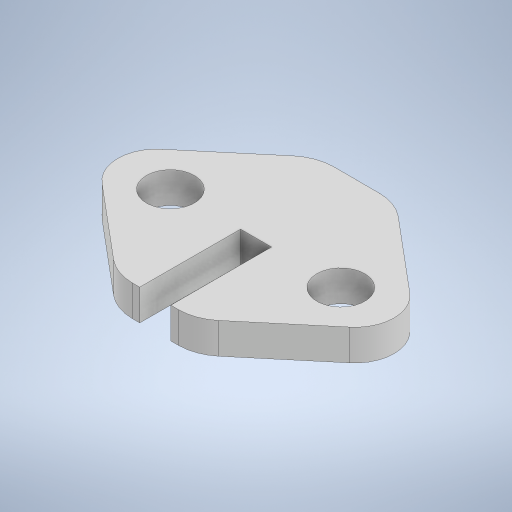
# Autodesk Inventor part: back_lock
Saved by Autodesk Inventor 2024 (Build 280153000, 153)
## iProperties
Created: 2024-04-22
Part Number: back_lock
Material: Generic
Document SubType Name: Modeling
Designer: nikop
Density: 1 g/cm^3
Appearance: Default
Author: nikop
Autodesk Inventor part; units mm, degrees
ref_plane "YZ Plane" through (0, 0, 0) normal (1, 0, 0) x (0, 1, 0)
ref_plane "XZ Plane" through (0, 0, 0) normal (0, 1, 0) x (-1, 0, 0)
ref_plane "XY Plane" through (0, 0, 0) normal (0, 0, 1) x (1, 0, 0)
sketch "Sketch1" plane through (0, 0, 0) normal (0, 1, 0) x (-1, 0, 0)
  line L0 (4.2489, -4.8935) -> (8.8452, -1.0368)
  line L1 (-0.6227, -5.5713) -> (0.8666, -5.5713)
  arc A0 (2.3695, -5.5775) -> (4.2489, -4.8935) centre (2.3418, -2.5777) ccw
  line L2 (0.8803, -5.5773) -> (2.3695, -5.5775)
  arc A1 (-2.502, -4.8873) -> (-0.6227, -5.5713) centre (-0.595, -2.5715) ccw
  circle A2 centre (6.3667, 0.9564) radius 1.55
  arc A3 (8.8452, -1.0368) -> (8.8476, 2.8817) centre (7.2935, 0.9234) ccw
  line L3 (-0.1334, 0.9212) -> (1.8666, 0.9212)
  arc A4 (-0.6442, 7.4287) -> (-2.5236, 6.7446) centre (-0.6165, 4.4288) ccw
  line L4 (-0.6442, 7.4287) -> (-0.1334, 7.4287)
  line L5 (-0.1334, 0.9212) -> (-0.1334, 7.4287)
  line L6 (1.8666, 0.9212) -> (1.8827, 7.4237)
  line L7 (1.8827, 7.4237) -> (2.372, 7.4225)
  arc A5 (4.2514, 6.7384) -> (2.372, 7.4225) centre (2.3443, 4.4226) ccw
  line L8 (4.2514, 6.7384) -> (8.8476, 2.8817)
  line L9 (-2.502, -4.8873) -> (-7.0983, -1.0306)
  line L10 (-2.5236, 6.7446) -> (-7.1199, 2.8879)
  circle A6 centre (-4.6336, 0.9477) radius 1.55
  arc A7 (-7.1199, 2.8879) -> (-7.0983, -1.0306) centre (-5.5563, 0.9372) ccw
  line L11 (0.8803, -5.5773) -> (0.8666, -5.5713)
  point P0 (0, 0)
  dimension "d0" = 2
  dimension "d1" = 3
  dimension "d2" = 2
  dimension "d3" = 3
  dimension "d4" = 2
  dimension "d5" = 3
  dimension "d6" = 2
  dimension "d7" = 3
  dimension "d8" = 3.1
  dimension "d9" = 3.1
  dimension "d10" = 6
  dimension "d11" = 6
  dimension "d12" = 2.5
  dimension "d13" = 6
  dimension "d14" = 6
  dimension "d15" = 2.5
  constraints: 24 end point, 12 point on circle, 8 centre point, 1 horizontal, 1 perpendicular
  measures "d0" distance of L7.end L8.start
  measures "d1" radius of A5
  measures "d2" distance of L2.end L0.start
  measures "d3" radius of A0
  measures "d4" distance of L4.start L10.start
  measures "d5" radius of A4
  measures "d6" distance of L1.start L9.start
  measures "d7" radius of A1
  measures "d8" diameter of A6
  measures "d9" diameter of A2
  measures "d10" distance of L10.start L10.end
  measures "d11" distance of L9.start L9.end
  measures "d12" radius of A7
  measures "d13" distance of L0.start L0.end
  measures "d14" distance of L8.start L8.end
  measures "d15" radius of A3
extrude "Extrusion1" add sketch "Sketch1" along normal blind 2
body "Solid1"
